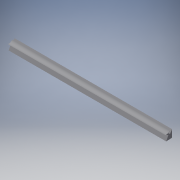
# Autodesk Inventor part: juncao tela - som
Saved by Autodesk Inventor 2016 (Build 200138000, 138)
## iProperties
Created: 2017-06-28
Part Number: juncao tela - som
Material: Genérico
Document SubType Name: Modeling
Designer: Fabio
Density: 1 g/cm^3
Appearance: Padrão
Author: Fabio
Autodesk Inventor part; units mm, degrees
ref_plane "YZ Plane" through (0, 0, 0) normal (1, 0, 0) x (0, 1, 0)
ref_plane "XZ Plane" through (0, 0, 0) normal (0, 1, 0) x (-1, 0, 0)
ref_plane "XY Plane" through (0, 0, 0) normal (0, 0, 1) x (1, 0, 0)
sketch "Esboço1" plane through (0, 0, 0) normal (1, 0, 0) x (0, 1, 0)
  line L0 (8.7685, 9.8534) -> (4.4419, 3.3376)
  line L1 (4.4419, 3.3376) -> (1.0821, 5.5685)
  line L2 (1.0821, 5.5685) -> (3.8705, 9.768)
  line L3 (-5.1511, 5.9928) -> (0.9304, 2.875)
  line L4 (0.9304, 2.875) -> (-3.5768, -6.1466)
  line L5 (8.7685, 9.8534) -> (8.7685, -5.5484)
  line L6 (8.7685, -5.5484) -> (-3.5905, -6.174)
  line L7 (-3.5905, -6.174) -> (-3.5768, -6.1466)
  arc A0 (-5.1511, 5.9928) -> (3.8705, 9.768) centre (-3.4697, 14.6419) ccw
  constraints: 16 end point, 2 perpendicular, 2 point on circle, 2 point on line, 1 centre point, 1 tangent, 1 vertical
extrude "Extrusão1" add sketch "Esboço1" along normal blind 330
